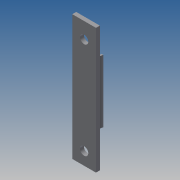
# Autodesk Inventor part: feedCableStay1
Saved by Autodesk Inventor 2014 SP1 (Build 180222100, 222)
## iProperties
Created: 2014-08-29
Part Number: feedCableStay1
Material: Generic
Document SubType Name: Modeling
Designer: Dave
Density: 1 g/cm^3
Appearance: Default
Author: Dave
Autodesk Inventor part; units mm, degrees
ref_plane "YZ Plane" through (0, 0, 0) normal (1, 0, 0) x (0, 1, 0)
ref_plane "XZ Plane" through (0, 0, 0) normal (0, 1, 0) x (-1, 0, 0)
sketch "Sketch1" plane through (0, 0, 0) normal (0, 1, 0) x (-1, 0, 0)
  arc A0 (6.35, 0) -> (-6.35, 0) centre (0, 0) ccw
  arc A1 (5.08, 0) -> (-5.08, 0) centre (0, 0) ccw
  line L0 (-6.35, 0) -> (-5.08, 0)
  line L1 (5.08, 0) -> (6.35, 0)
  dimension "d0" = 12.7
  dimension "d1" = 1.27
  constraints: 4 end point, 4 point on circle, 2 centre point, 2 horizontal, 1 coincident
  measures "d0" diameter of A0
  measures "d1" radial gap between concentric circles of A1 A0
extrude "Extrusion1" add sketch "Sketch1" along normal blind 50.8
sketch "Sketch2" plane through (0, 50.8, 0) normal (0, 1, 0) x (1, 0, 0)
  arc A0 (-6.35, 0) -> (6.35, 0) centre (0, 0) ccw projected
  line L0 (6.35, 0) -> (5.08, 0) projected
  arc A1 (-5.08, 0) -> (5.08, 0) centre (0, 0) ccw projected
  line L1 (-5.08, 0) -> (-6.35, 0) projected
  point P0 (0, -6.35)
  constraints: 1 point on circle
ref_plane "Work Plane1" through (0, 50.8, 6.35) normal (0, 0, 1) x (1, 0, 0)
sketch "Sketch3" plane through (0, 50.8, 6.35) normal (0, 0, 1) x (1, 0, 0)
  line L0 (-9.2332, -76.1134) -> (9.971, -76.1134)
  line L1 (9.971, -76.1134) -> (9.971, 25.4866)
  line L2 (9.971, 25.4866) -> (-9.2332, 25.4866)
  line L3 (-9.2332, 25.4866) -> (-9.2332, -76.1134)
  point P0 (0, -50.8)
  dimension "d4" = 101.6
  constraints: 8 end point, 2 parallel, 1 horizontal, 1 perpendicular
  measures "d4" distance of L1.end L0.end
extrude "Extrusion2" add sketch "Sketch3" along normal blind 3.175
sketch "Sketch4" plane through (0, 50.8, 6.35) normal (0, 0, -1) x (-1, 0, 0)
  circle A0 centre (-0.3689, 12.6095) radius 2.8969
  circle A1 centre (-0.3689, -65.6928) radius 3.2786
  constraints: 2 centre point
hole "Hole1" at (0.3689, 63.4095, 6.35) at (0.3689, -14.8928, 6.35) direction (0, 0, 1) diameter 6.7564 end through all clearance for "Flat Head Machine Screw (82)" size "1/4" standard "Ansi Unified Screw Threads"
body "Solid1"
